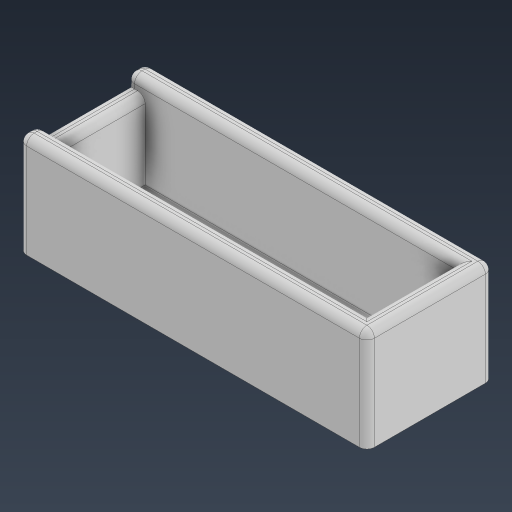
# Autodesk Inventor part: battery_compartment
Saved by Autodesk Inventor 2024 (Build 280153000, 153)
## iProperties
Created: 2024-07-25
Part Number: battery_compartment
Material: Generic
Document SubType Name: Modeling
Designer: Piter
Density: 1 g/cm^3
Appearance: Default
Author: Piter
Autodesk Inventor part; units mm, degrees
ref_plane "YZ Plane" through (0, 0, 0) normal (1, 0, 0) x (0, 1, 0)
ref_plane "XZ Plane" through (0, 0, 0) normal (0, 1, 0) x (-1, 0, 0)
ref_plane "XY Plane" through (0, 0, 0) normal (0, 0, 1) x (1, 0, 0)
sketch "Sketch1" plane through (0, 0, 0) normal (0, 1, 0) x (-1, 0, 0)
  line L0 (0, 0) -> (52, 0)
  line L1 (52, 0) -> (52, -15)
  line L2 (52, -15) -> (0, -15)
  line L3 (0, -15) -> (0, 0)
  line L4 (55, 3) -> (-3, 3)
  line L5 (-3, 3) -> (-3, -18)
  line L6 (-3, -18) -> (55, -18)
  line L7 (55, -18) -> (55, 3)
  dimension "d0" = 52
  dimension "d1" = 15
  dimension "d2" = 3
  dimension "d3" = 3
  dimension "d4" = 3
  dimension "d5" = 3
  constraints: 16 end point, 4 parallel, 2 horizontal, 2 perpendicular
  measures "d0" distance of L1.end L2.end
  measures "d1" distance of L0.end L1.end
  measures "d2" distance between parallel lines of L6 L2
  measures "d3" distance between parallel lines of L4 L0
  measures "d4" distance between parallel lines of L1 L7
  measures "d5" distance between parallel lines of L5 L3
extrude "Extrusion1" add sketch "Sketch1" along normal blind 2 contours L0 L1 L2 L3
extrude "Extrusion2" add sketch "Sketch1" along normal blind 17
sketch "Sketch2" plane through (0, 17, 0) normal (0, 1, 0) x (1, 0, 0)
  line L0 (-52, 15) -> (0, 15) projected
  line L1 (-55, 18) -> (-55, -3) projected
  line L2 (-52, 15) -> (-55, 15)
  line L3 (-55, 15) -> (-55, 0)
  line L4 (-55, 0) -> (-52, 0)
  line L5 (-52, 0) -> (-52, 15)
  point P0 (0, 0)
  constraints: 8 end point, 2 parallel, 1 horizontal, 1 perpendicular, 1 point on line
extrude "Extrusion3" cut sketch "Sketch2" against normal blind 2
fillet "Fillet1" radius 1.25 10 edges at (-27.5, 17, -15) (-27.5, 17, 0) (-26, 17, -18) (-26, 17, 3) (0, 17, -7.5) (3, 17, -7.5) (-55, 15, -7.5) (-52, 15, -7.5) (-55, 16, -15) (-55, 16, 0)
fillet "Fillet2" radius 1.25 12 edges at (-55, 16.6339, 2.6339) (-55, 17, 1.5) (-54.6339, 16.6339, 0.3661) (-55, 7.875, 3) (-55, 16.6339, -17.6339) (-55, 17, -16.5) (-54.6339, 16.6339, -15.3661) (-55, 7.875, -18) (2.6339, 16.6339, 2.6339) (3, 7.875, 3) (2.6339, 16.6339, -17.6339) (3, 7.875, -18)
body "Solid1"
